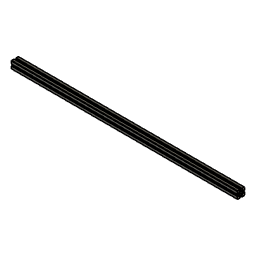
8020 4040 Aluminum v2 (Autodesk Fusion 360 design; units mm, degrees)
Autodesk Fusion 360 part; units mm, degrees
sketch "Sketch1" plane through (0, 0, 0) normal (1, 0, 0) x (0, 1, 0)
  circle A0 centre (0, 0) radius 3.405
  line L0 (3.7374, -7.6205) -> (-3.7051, -7.6205)
  line L1 (-3.7051, 7.5882) -> (3.7325, 7.5882)
  line L2 (7.425, -7.6205) -> (-7.425, 7.6205) construction
  line L3 (-7.425, -7.6205) -> (2.3762, 2.4388) construction
  line L4 (20, -20) -> (-20, 20) construction
  line L5 (15.425, -15.6205) -> (-15.425, 15.6205) construction
  line L6 (-8.0311, -5.0519) -> (-12.0311, -9.0087)
  line L7 (16.9453, -20) -> (68.4291, -20) construction
  line L8 (5.1526, 8.18) -> (9.3917, 12.4549)
  line L9 (-5.1193, 8.174) -> (-9.1412, 12.1959)
  line L10 (12.0634, -9.0087) -> (8.2063, -5.1516)
  line L11 (8.2063, 5.1193) -> (12.0634, 8.9764)
  line L12 (-9.1412, -12.2283) -> (-5.1193, -8.2063)
  line L13 (9.1735, -12.2283) -> (5.1516, -8.2063)
  line L14 (-8.0638, 5.2264) -> (-12.0311, 8.9764)
  line L15 (-20, -20) -> (2.4077, 2.4077) construction
  line L16 (7.425, 7.425) -> (20, 20) construction
  line L17 (-15.425, -15.6205) -> (2.3925, 2.4228) construction
  line L18 (7.6205, 3.7051) -> (7.6205, -3.7374)
  line L19 (-7.4376, -3.6301) -> (-7.4376, 3.7729)
  line L20 (-19, -4.065) -> (-16.4376, -4.065)
  line L21 (-16.4376, 4.065) -> (-19, 4.065)
  line L22 (16.47, 4.065) -> (19, 4.065)
  line L23 (19, -4.065) -> (16.47, -4.065)
  line L24 (-20, -18) -> (-20, -5.065)
  line L25 (-20, 5.065) -> (-20, 18)
  line L26 (-15.4376, -7.5869) -> (-15.4376, -5.065)
  line L27 (-15.4376, 5.065) -> (-15.4376, 7.5546)
  line L28 (15.47, 7.5546) -> (15.47, 5.065)
  line L29 (15.47, -5.065) -> (15.47, -7.5869)
  line L30 (20, 18) -> (20, 5.065)
  line L31 (20, -5.065) -> (20, -18)
  line L32 (16.47, 4.065) -> (19, 4.065)
  line L33 (4.065, 19) -> (4.065, 16.5882)
  line L34 (-4.065, 16.5882) -> (-4.065, 19)
  line L35 (4.065, -19) -> (4.065, -16.6205)
  line L36 (-4.065, -16.6205) -> (-4.065, -19)
  line L37 (-7.7361, 15.5882) -> (-5.065, 15.5882)
  line L38 (5.065, 15.5882) -> (7.7684, 15.5882)
  line L39 (-18, 20) -> (-5.065, 20)
  line L40 (5.065, 20) -> (18, 20)
  line L41 (-16.9453, -20) -> (-5.065, -20) construction
  line L42 (5.065, -20) -> (34.3692, -20) construction
  line L43 (18, -20) -> (4.065, -20)
  line L44 (-4.065, -20) -> (-18, -20)
  line L45 (7.7684, -15.6205) -> (5.065, -15.6205)
  line L46 (-5.065, -15.6205) -> (-7.7361, -15.6205)
  arc A1 (-18, 20) -> (-20, 18) centre (-18, 18) ccw
  arc A2 (20, 18) -> (18, 20) centre (18, 18) ccw
  arc A3 (18, -20) -> (20, -18) centre (18, -18) ccw
  arc A4 (-20, -18) -> (-18, -20) centre (-18, -18) ccw
  arc A5 (-9.1412, -12.2283) -> (-7.7361, -15.6205) centre (-7.7361, -13.6334) ccw
  arc A6 (-15.4376, -7.5869) -> (-12.0311, -9.0087) centre (-13.4376, -7.5869) ccw
  arc A7 (7.7684, -15.6205) -> (9.1735, -12.2283) centre (7.7684, -13.6334) ccw
  arc A8 (12.0634, -9.0087) -> (15.47, -7.5869) centre (13.47, -7.5869) ccw
  arc A9 (-12.0311, 8.9764) -> (-15.4376, 7.5546) centre (-13.4376, 7.5546) ccw
  arc A10 (-7.7361, 15.5882) -> (-9.1412, 12.1959) centre (-7.7361, 13.6011) ccw
  arc A11 (9.1735, 12.1959) -> (7.7684, 15.5882) centre (7.7684, 13.6011) ccw
  arc A12 (15.47, 7.5546) -> (12.0634, 8.9764) centre (13.47, 7.5546) ccw
  arc A13 (16.47, -4.065) -> (15.47, -5.065) centre (16.47, -5.065) ccw
  arc A14 (20, -5.065) -> (19, -4.065) centre (19, -5.065) ccw
  arc A15 (5.065, -15.6205) -> (4.065, -16.6205) centre (5.065, -16.6205) ccw
  arc A16 (4.065, -19) -> (5.065, -20) centre (5.065, -19) ccw
  arc A17 (-4.065, -16.6205) -> (-5.065, -15.6205) centre (-5.065, -16.6205) ccw
  arc A18 (-5.065, -20) -> (-4.065, -19) centre (-5.065, -19) ccw
  arc A19 (-19, -4.065) -> (-20, -5.065) centre (-19, -5.065) ccw
  arc A20 (-15.4376, -5.065) -> (-16.4376, -4.065) centre (-16.4376, -5.065) ccw
  arc A21 (-20, 5.065) -> (-19, 4.065) centre (-19, 5.065) ccw
  arc A22 (-16.4376, 4.065) -> (-15.4376, 5.065) centre (-16.4376, 5.065) ccw
  arc A23 (-4.065, 19) -> (-5.065, 20) centre (-5.065, 19) ccw
  arc A24 (-5.065, 15.5882) -> (-4.065, 16.5882) centre (-5.065, 16.5882) ccw
  arc A25 (4.065, 16.5882) -> (5.065, 15.5882) centre (5.065, 16.5882) ccw
  arc A26 (5.065, 20) -> (4.065, 19) centre (5.065, 19) ccw
  arc A27 (15.47, 5.065) -> (16.47, 4.065) centre (16.47, 5.065) ccw
  arc A28 (19, 4.065) -> (20, 5.065) centre (19, 5.065) ccw
  arc A29 (3.7325, 7.5882) -> (5.1526, 8.18) centre (3.7325, 9.5882) ccw
  arc A30 (8.2063, 5.1193) -> (7.6205, 3.7051) centre (9.6205, 3.7051) ccw
  arc A31 (7.6205, -3.7374) -> (8.2063, -5.1516) centre (9.6205, -3.7374) ccw
  arc A32 (5.1516, -8.2063) -> (3.7374, -7.6205) centre (3.7374, -9.6205) ccw
  arc A33 (-3.7051, -7.6205) -> (-5.1193, -8.2063) centre (-3.7051, -9.6205) ccw
  arc A34 (-8.0311, -5.0519) -> (-7.4376, -3.6301) centre (-9.4376, -3.6301) ccw
  arc A35 (-7.4376, 3.7729) -> (-8.0638, 5.2264) centre (-9.4376, 3.7729) ccw
  arc A36 (-5.1193, 8.174) -> (-3.7051, 7.5882) centre (-3.7051, 9.5882) ccw
  dimension "d1" = 6.81
  dimension "d4" = 40
  dimension "d5" = 40
  dimension "d7" = 8
  dimension "d9" = 45
  dimension "d11" = 135
  dimension "d12" = 4.32
  dimension "d13" = 2.16
  dimension "d16" = 8.13
  dimension "d17" = 2
  dimension "d18" = 2
  dimension "d19" = 2
  dimension "d20" = 2
  dimension "d22" = 2
  dimension "d23" = 8
  dimension "d24" = 8
  dimension "d26" = 1
  dimension "d27" = 1
  dimension "d28" = 1
  dimension "d29" = 1
  dimension "d30" = 1
  dimension "d31" = 1
  dimension "d32" = 1
  dimension "d33" = 1
  dimension "d34" = 1
  dimension "d35" = 1
  dimension "d36" = 1
  dimension "d37" = 1
  dimension "d38" = 1
  dimension "d39" = 1
  dimension "d40" = 1
  dimension "d41" = 1
  dimension "d42" = 8.13
  dimension "d43" = 8.13
  dimension "d44" = 8.13
  dimension "d45" = 2
  dimension "d46" = 2
  dimension "d47" = 2
  dimension "d48" = 2
  dimension "d49" = 2
  dimension "d50" = 2
  dimension "d51" = 2
  dimension "d52" = 2
  constraint coincident A0.centre origin
  constraint horizontal L0
  constraint parallel L0 L1
  constraint coincident L2 A0.centre
  constraint coincident L3 A0.centre
  constraint horizontal L43
  constraint perpendicular L24 L43
  constraint parallel L39 L43
  constraint parallel L24 L30
  constraint coincident L4 A0.centre
  constraint coincident A0.centre L15
  constraint horizontal L45
  constraint parallel L37 L45
  constraint coincident L5 A0.centre
  constraint coincident A0.centre L17
  constraint horizontal L41
  constraint coincident L41.start L43
  constraint horizontal L7
  constraint coincident L7.start L43
  constraint parallel L10 L13
  constraint collinear L9 L10
  constraint collinear L11 L12
  constraint coincident L16.start L15
  constraint coincident A0 L15.end
  constraint collinear L15 L16
  constraint coincident A0 L17.end
  constraint coincident A0 L3.end
  constraint horizontal L20
  constraint horizontal L21
  constraint collinear L24 L25
  constraint collinear L26 L27
  constraint collinear L28 L29
  constraint collinear L30 L31
  constraint vertical L33
  constraint vertical L34
  constraint collinear L37 L38
  constraint collinear L39 L40
  constraint collinear L41 L42
  constraint collinear L43 L44
  constraint collinear L45 L46
  constraint parallel L18 L19
  constraint coincident L4.end L25
  constraint coincident L4.end L39
  constraint tangent L25 A1
  constraint tangent L39 A1
  constraint coincident L16.end L40
  constraint tangent L40 A2
  constraint tangent L30 A2
  constraint coincident L4.start L31
  constraint coincident L4.start L43
  constraint tangent L31 A3
  constraint tangent L43 A3
  constraint coincident L15.start L44
  constraint coincident L15.start L24
  constraint tangent L44 A4
  constraint tangent L24 A4
  constraint tangent L12 A5
  constraint tangent L46 A5
  constraint tangent L6 A6
  constraint tangent L26 A6
  constraint coincident A11 L8.end
  constraint tangent L29 A13
  constraint tangent L23 A13
  constraint tangent L23 A14
  constraint tangent L31 A14
  constraint tangent L45 A15
  constraint tangent L35 A15
  constraint coincident L43.end L35
  constraint tangent L35 A16
  constraint tangent L42 A16
  constraint tangent L46 A17
  constraint tangent L36 A17
  constraint coincident L44.start L36
  constraint tangent L41 A18
  constraint tangent L36 A18
  constraint tangent L24 A19
  constraint tangent L20 A19
  constraint tangent L20 A20
  constraint tangent L26 A20
  constraint tangent L25 A21
  constraint tangent L21 A21
  constraint tangent L21 A22
  constraint tangent L27 A22
  constraint tangent L39 A23
  constraint tangent L34 A23
  constraint tangent L37 A24
  constraint tangent L34 A24
  constraint tangent L33 A25
  constraint tangent L38 A25
  constraint tangent L33 A26
  constraint tangent L40 A26
  constraint tangent L28 A27
  constraint tangent L32 A27
  constraint tangent L22 A28
  constraint tangent L30 A28
  constraint tangent L1 A29
  constraint tangent L8 A29
  constraint tangent L11 A30
  constraint tangent L18 A30
  constraint tangent L18 A31
  constraint tangent L10 A31
  constraint tangent L0 A32
  constraint tangent L13 A32
  constraint tangent L12 A33
  constraint tangent L0 A33
  constraint tangent L6 A34
  constraint tangent L19 A34
  constraint tangent L14 A35
  constraint tangent L19 A35
  constraint tangent L9 A36
  constraint tangent L1 A36
  measures "d1" diameter of A0
  measures "d4" distance of L4.end L16.end
  measures "d5" distance of L15.start L4.end
  measures "d7" distance of L1 L37
  measures "d9" angle of L12 L41
  measures "d11" angle of L7 L13
  measures "d12" distance of L10 L13
  measures "d13" distance of L4 L13
  measures "d16" distance of L33 L34
  measures "d17" radius of A1
  measures "d18" radius of A2
  measures "d19" radius of A3
  measures "d20" radius of A4
  measures "d22" radius of A6
  measures "d23" distance of L19 L26
  measures "d24" distance of L0 L45
  measures "d26" radius of A13
  measures "d27" radius of A14
  measures "d28" radius of A15
  measures "d29" radius of A16
  measures "d30" radius of A17
  measures "d31" radius of A18
  measures "d32" radius of A19
  measures "d33" radius of A20
  measures "d34" radius of A21
  measures "d35" radius of A22
  measures "d36" radius of A23
  measures "d37" radius of A24
  measures "d38" radius of A25
  measures "d39" radius of A26
  measures "d40" radius of A27
  measures "d41" radius of A28
  measures "d42" distance of L20 L21
  measures "d43" distance of L23 L32
  measures "d44" distance of L35 L36
  measures "d45" radius of A29
  measures "d46" radius of A30
  measures "d47" radius of A31
  measures "d48" radius of A32
  measures "d49" radius of A33
  measures "d50" radius of A34
  measures "d51" radius of A35
  measures "d52" radius of A36
extrude "Extrude1" add sketch "Sketch1" along normal blind 1219.2
equation "d13 = ( 4.32 / 2 ) * 1 mm"
